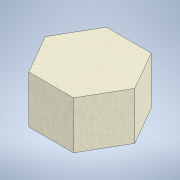
# Autodesk Inventor part: Hex_Blues
Saved by Autodesk Inventor 2021 (Build 250183000, 183)
## iProperties
Created: 2023-03-16
Part Number: Hex_Blues
Material: Paper
Document SubType Name: Modeling
Designer: Bradley
Density: 0.93 g/cm^3
Appearance: Cardboard - Chipboard
Author: Bradley
Autodesk Inventor part; units mm, degrees
ref_plane "YZ Plane" through (0, 0, 0) normal (1, 0, 0) x (0, 1, 0)
ref_plane "XZ Plane" through (0, 0, 0) normal (0, 1, 0) x (-1, 0, 0)
ref_plane "XY Plane" through (0, 0, 0) normal (0, 0, 1) x (1, 0, 0)
sketch "Sketch1" plane through (0, 0, 0) normal (0, 1, 0) x (-1, 0, 0)
  line L0 (-29.1562, -50.5) -> (-58.3124, 0)
  line L1 (-58.3124, 0) -> (-29.1562, 50.5)
  line L2 (-29.1562, 50.5) -> (29.1562, 50.5)
  line L3 (29.1562, 50.5) -> (58.3124, 0)
  line L4 (58.3124, 0) -> (29.1562, -50.5)
  line L5 (29.1562, -50.5) -> (-29.1562, -50.5)
  point P0 (0, 0)
  point P1 (0, 0)
  dimension "d0" = 101
  constraints: 12 end point, 1 coincident, 1 horizontal, 13 other
  measures "d0" distance between parallel lines of L2 L5
extrude "Extrusion1" add sketch "Sketch1" along normal mid plane 62
body "Solid1"
